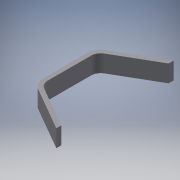
# Autodesk Inventor part: nozzle mask back
Saved by Autodesk Inventor 2016 SP1 (Build 200210100, 210)
## iProperties
Created: 2016-04-21
Part Number: nozzle mask back
Material: Generic
Document SubType Name: Modeling
Designer: ubik
Density: 1 g/cm^3
Appearance: Default
Author: ubik
Autodesk Inventor part; units mm, degrees
ref_plane "YZ Plane" through (0, 0, 0) normal (1, 0, 0) x (0, 1, 0)
ref_plane "XZ Plane" through (0, 0, 0) normal (0, 1, 0) x (-1, 0, 0)
ref_plane "XY Plane" through (0, 0, 0) normal (0, 0, 1) x (1, 0, 0)
sketch "Sketch1" plane through (0, 0, 0) normal (0, 0, 1) x (1, 0, 0)
  circle A0 centre (-21.75, -3) radius 1 projected
  circle A1 centre (-20, 14) radius 1.5 projected
  circle A2 centre (-20, -14) radius 1.5 projected
  circle A3 centre (21, 8.5) radius 1.5 projected
  circle A4 centre (9, 0) radius 1.5 projected
  circle A5 centre (21, -8.5) radius 1.5
  circle A6 centre (12, -9) radius 6
  circle A7 centre (12, 9) radius 6 projected
  circle A8 centre (5.9186, 35.7487) radius 2 projected
  circle A9 centre (5.9186, -35.7487) radius 2 projected
  circle A10 centre (28, -23) radius 2 projected
  circle A11 centre (28, 23) radius 2 projected
  arc A12 (34, 23) -> (31, 28.1962) centre (28, 23) ccw projected
  line L0 (31, 28.1962) -> (8.9186, 40.9449) projected
  arc A13 (8.9186, 40.9449) -> (2.9186, 40.9449) centre (5.9186, 35.7487) ccw projected
  arc A14 (2.9186, -40.9449) -> (8.9186, -40.9449) centre (5.9186, -35.7487) ccw projected
  line L1 (8.9186, -40.9449) -> (31, -28.1962) projected
  arc A15 (31, -28.1962) -> (34, -23) centre (28, -23) ccw projected
  line L2 (34, -23) -> (34, 23) projected
  line L3 (-12.8721, -31.2507) -> (-12.8721, -34.1375)
  line L4 (-12.8721, 34.1375) -> (-12.8721, 31.2507)
  line L5 (-36.6686, 17.5119) -> (-12.8721, 31.2507)
  arc A16 (-39.4186, -12.7487) -> (-36.6686, -17.5119) centre (-33.9186, -12.7487) ccw
  line L6 (-39.4186, -12.7487) -> (-39.4186, 12.7487)
  arc A17 (-36.6686, 17.5119) -> (-39.4186, 12.7487) centre (-33.9186, 12.7487) ccw
  line L7 (-37.9186, 19.6769) -> (-12.8721, 34.1375)
  arc A18 (-41.9186, -12.7487) -> (-37.9186, -19.6769) centre (-33.9186, -12.7487) ccw
  line L8 (-41.9186, -12.7487) -> (-41.9186, 12.7487)
  arc A19 (-37.9186, 19.6769) -> (-41.9186, 12.7487) centre (-33.9186, 12.7487) ccw
  arc A20 (-36.6686, 17.5119) -> (-39.4186, 12.7487) centre (-33.9186, 12.7487) ccw
  arc A21 (-39.4186, -12.7487) -> (-36.6686, -17.5119) centre (-33.9186, -12.7487) ccw
  line L9 (-12.8721, -34.1375) -> (-37.9186, -19.6769)
  line L10 (-12.8721, -31.2507) -> (-36.6686, -17.5119)
  constraints: 16 end point, 12 point on circle, 8 centre point, 2 tangent
extrude "Extrusion1" add sketch "Sketch1" along normal blind 10 contours L3 L9 A18 L8 A19 L7 L4 L5 A17 L6 A16 L10
body "Solid1"
